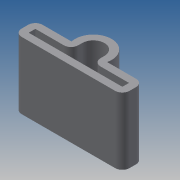
# Autodesk Inventor part: ribbon cable management
Saved by Autodesk Inventor 2013 (Build 170138000, 138)
## iProperties
Created: 2017-04-10
Part Number: ribbon cable management
Material: Generic
Document SubType Name: Modeling
Designer: employee
Density: 1 g/cm^3
Author: employee
Autodesk Inventor part; units mm, degrees
ref_plane "YZ Plane" through (0, 0, 0) normal (1, 0, 0) x (0, 1, 0)
ref_plane "XZ Plane" through (0, 0, 0) normal (0, 1, 0) x (-1, 0, 0)
ref_plane "XY Plane" through (0, 0, 0) normal (0, 0, 1) x (1, 0, 0)
sketch "Sketch1" plane through (0, 0, 0) normal (0, 0, 1) x (1, 0, 0)
  line L0 (-10.5, 0.75) -> (10.5, 0.75)
  line L1 (10.5, 0.75) -> (10.5, -0.75)
  line L2 (10.5, -0.75) -> (-10.5, -0.75)
  line L3 (-10.5, -0.75) -> (-10.5, 0.75)
  circle A0 centre (0, 3.25) radius 2.5
  arc A1 (4, 2.35) -> (-4, 2.35) centre (0, 3.25) ccw
  line L4 (-12.1, 2.35) -> (-12.1, -2.35)
  line L5 (-12.1, -2.35) -> (12.1, -2.35)
  line L6 (12.1, -2.35) -> (12.1, 2.35)
  line L7 (12.1, 2.35) -> (4, 2.35)
  line L8 (-4, 2.35) -> (-12.1, 2.35)
  line L9 (-2.5, 3.25) -> (-2.5, 0.75)
  line L10 (2.5, 3.25) -> (2.5, 0.75)
  point P0 (0, 0)
  point P1 (-10.5, 0)
  point P2 (10.5, 0)
  point P3 (0, 0.75)
  dimension "d0" = 1.5
  dimension "d2" = 21
  dimension "d3" = 5
  dimension "d4" = 1.6
  dimension "d5" = 1.6
  dimension "d6" = 1.6
  dimension "d7" = 1.6
  constraints: 22 end point, 5 parallel, 5 perpendicular, 4 point on circle, 3 midpoint, 3 tangent, 2 centre point, 2 horizontal alignment, 2 point on line, 2 vertical alignment, 1 horizontal, 2 other
  measures "d0" distance between parallel lines of L2 L0
  measures "d2" distance of L1.end L2.end
  measures "d3" diameter of A0
  measures "d4" radial gap between concentric circles of A1 A0
  measures "d5" distance between parallel lines of L8 L0
  measures "d6" distance between parallel lines of L4 L3
  measures "d7" distance between parallel lines of L7 L0
extrude "Extrusion1" add sketch "Sketch1" along normal blind 15
fillet "Fillet1" radius 1.6 6 edges at (-2.5, 0.75, 7.5) (2.5, 0.75, 7.5) (12.1, -2.35, 7.5) (12.1, 2.35, 7.5) (-12.1, -2.35, 7.5) (-12.1, 2.35, 7.5)
body "Solid1"
